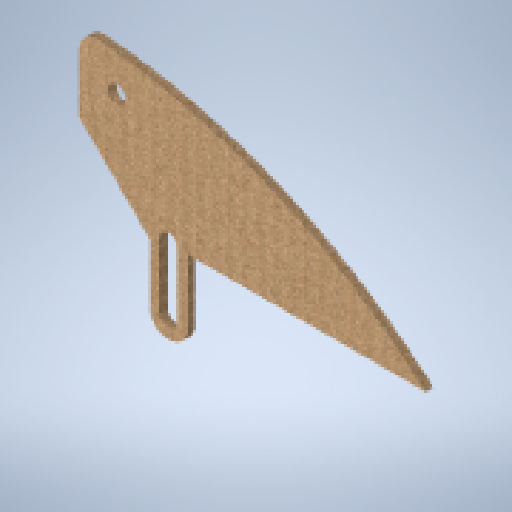
# Autodesk Inventor part: Dedo-BC
Saved by Autodesk Inventor 2023.1 (Build 271208000, 208)
## iProperties
Created: 2022-11-11
Part Number: Dedo-BC
Material: MDF Medium Density Fiberboard
Document SubType Name: Modeling
Designer: Daniel Peña
Density: 0.8 g/cm^3
Appearance: Cardboard - Corrugated
Author: Daniel Peña
Autodesk Inventor part; units mm, degrees
ref_plane "YZ Plane" through (0, 0, 0) normal (1, 0, 0) x (0, 1, 0)
ref_plane "XZ Plane" through (0, 0, 0) normal (0, 1, 0) x (-1, 0, 0)
ref_plane "XY Plane" through (0, 0, 0) normal (0, 0, 1) x (1, 0, 0)
sketch "Sketch1" plane through (0, 0, 0) normal (0, 0, 1) x (1, 0, 0)
  line L0 (7.5, 0) -> (7.5, -25)
  line L1 (0, -32.5) -> (0, -32.5)
  line L2 (-7.5, -25) -> (-7.5, -2.139)
  line L3 (0, 0) -> (0, -25) construction
  arc A0 (-7.5, -25) -> (0, -32.5) centre (0, -25) ccw
  arc A1 (0, -32.5) -> (7.5, -25) centre (0, -25) ccw
  line L4 (0, -28.5) -> (0, -28.5)
  line L5 (-3.5, -25) -> (-3.5, 0)
  line L6 (0, 3.5) -> (0, 3.5)
  line L7 (3.5, 0) -> (3.5, -25)
  arc A2 (-3.5, -25) -> (0, -28.5) centre (0, -25) ccw
  arc A3 (0, -28.5) -> (3.5, -25) centre (0, -25) ccw
  arc A4 (3.5, 0) -> (0, 3.5) centre (0, 0) ccw
  arc A5 (0, 3.5) -> (-3.5, 0) centre (0, 0) ccw
  line L8 (7.5, 0) -> (100, 0)
  line L9 (-35, 25.361) -> (-35, 47.5)
  line L10 (-7.5, -2.139) -> (-35, 25.361)
  line L11 (-7.5, -2.139) -> (31.3909, -2.139) construction
  arc A6 (-27.5, 55) -> (-35, 47.5) centre (-27.5, 47.5) ccw
  arc A7 (100, 0) -> (-27.5, 55) centre (-45.2542, -161.4415) ccw
  point P0 (0, 0)
  point P1 (-20, 40)
  point P2 (0, -28.5)
  point P3 (0, 3.5)
  point P4 (0, -32.5)
  dimension "d0" = 20
  dimension "d2" = 25
  dimension "d8" = 15
  dimension "d9" = 7.5
  dimension "d10" = 7.5
  dimension "d11" = 3.5
  dimension "d12" = 3.5
  dimension "d13" = 7
  dimension "d14" = 3.5
  dimension "d28" = 40
  dimension "d30" = 135
  dimension "d31" = 15
  dimension "d33" = 7.5
  dimension "d34" = 120
  dimension "d35" = 217.1685
  dimension "d36" = 27.5
  constraints: 24 end point, 16 point on circle, 13 tangent, 8 centre point, 4 equal radius, 3 horizontal, 3 parallel, 1 coincident, 1 equal length, 1 perpendicular, 1 vertical, 2 other
  measures "d0" horizontal distance of L3.start point (-20, 40)
  measures "d2" distance of point (0, 0) L3.end
  measures "d8" distance between parallel lines of L0 L2
  measures "d9" distance from line of L3.end L1
  measures "d10" radius of A0
  measures "d11" distance from line of L6 point (0, 0)
  measures "d12" distance from line of L3.end L4
  measures "d13" distance between parallel lines of L7 L5
  measures "d14" radius of A2
  measures "d28" vertical distance of L3.start point (-20, 40)
  measures "d30" angle of L11 L10
  measures "d31" distance from line of point (-20, 40) L9
  measures "d33" radius of A6
  measures "d34" horizontal distance of L8.end point (-20, 40)
  measures "d35" radius of A7
  measures "d36" horizontal distance of L2.end L9.start
extrude "Extrusion1" add sketch "Sketch1" along normal blind 3
sketch "Sketch3" plane through (0, 0, 3) normal (0, 0, 1) x (1, 0, 0)
  arc A0 (-27.7773, 74.9035) -> (-35, 67.9071) centre (-28, 67.9071) ccw projected
  point P0 (0, 0)
  point P1 (-20, 40)
  dimension "d26" = 20
  dimension "d27" = 40
  measures "d26" horizontal distance of point (0, 0) point (-20, 40)
  measures "d27" vertical distance of point (0, 0) point (-20, 40)
hole "Hole1" at (-20, 40, 3) direction (0, 0, -1) diameter 7 end through all
body "Solid1"
